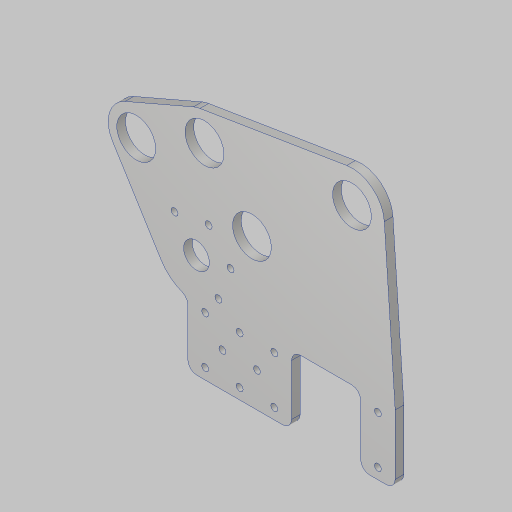
# Autodesk Inventor part: CL3-016
Saved by Autodesk Inventor 2023.5 (Build 275446000, 446)
## iProperties
Created: 2025-01-28
Part Number: CL3-016
Material: Aluminum 6061
Document SubType Name: Modeling
Designer: slick
Density: 2.7 g/cm^3
Appearance: Aluminum - Flat
Mass: 311.171 g
Surface Area: 423.623 cm^2
Volume: 115.249 cm^3
Author: slick
Autodesk Inventor part; units mm, degrees
ref_plane "YZ Plane" through (0, 0, 0) normal (1, 0, 0) x (0, 1, 0)
ref_plane "XZ Plane" through (0, 0, 0) normal (0, 1, 0) x (-1, 0, 0)
ref_plane "XY Plane" through (0, 0, 0) normal (0, 0, 1) x (1, 0, 0)
sketch "Sketch1" plane through (0, 0, 0) normal (0, 0, 1) x (1, 0, 0)
  line L0 (-76.2, 25.4) -> (76.2, 25.4) construction
  line L1 (76.2, 25.4) -> (76.2, -25.4) construction
  line L2 (76.2, -25.4) -> (-76.2, -25.4) construction
  line L3 (-76.2, -25.4) -> (-76.2, 25.4) construction
  line L4 (-76.2, 25.4) -> (76.2, -25.4) construction
  line L5 (76.2, 25.4) -> (-76.2, -25.4) construction
  line L6 (63.5, 17.4625) -> (63.5, -17.4625) construction
  line L7 (9.525, 15.875) -> (41.275, 15.875) construction
  line L8 (41.275, 15.875) -> (41.275, -15.875) construction
  line L9 (41.275, -15.875) -> (9.525, -15.875) construction
  line L10 (9.525, -15.875) -> (9.525, 15.875) construction
  line L11 (9.525, 15.875) -> (41.275, -15.875) construction
  line L12 (41.275, 15.875) -> (9.525, -15.875) construction
  line L13 (76.2, 101.6) -> (187.452, 101.6) construction
  line L14 (187.452, 101.6) -> (187.452, -25.4) construction
  line L15 (187.452, -25.4) -> (76.2, -25.4) construction
  line L16 (76.2, -25.4) -> (76.2, 101.6) construction
  line L17 (76.2, 101.6) -> (187.452, -25.4) construction
  line L18 (187.452, 101.6) -> (76.2, -25.4) construction
  point P0 (0, 0)
  point P1 (63.5, 0)
  point P2 (25.4, 0)
  point P3 (50.8, 0)
  point P4 (0, 0)
  point P5 (9.525, 0)
  point P6 (-12.7, 17.4625)
  point P7 (-12.7, -17.4625)
  point P8 (-25.4, 0)
  point P9 (-38.1, 17.4625)
  point P10 (-38.1, -17.4625)
  point P11 (-50.8, 0)
  point P12 (-63.5, 17.4625)
  point P13 (-63.5, -17.4625)
  point P14 (131.826, 38.1)
  dimension "d0" = 152.4
  dimension "d1" = 50.8
  dimension "d2" = 34.925
  dimension "d3" = 12.7
  dimension "d4" = 31.75
  dimension "d5" = 31.75
  dimension "d6" = 34.925
  dimension "d7" = 25.4
  dimension "d8" = 9.525
  dimension "d9" = 12.7
  dimension "d10" = 12.7
  dimension "d11" = 12.7
  dimension "d12" = 12.7
  dimension "d13" = 12.7
  dimension "d14" = 111.252
  dimension "d15" = 127
  dimension "d16" = 76.2
  constraints: 38 end point, 11 horizontal alignment, 8 midpoint, 6 parallel, 4 vertical alignment, 3 horizontal, 3 perpendicular, 2 coincident, 1 vertical
  measures "d0" distance of L1.end L2.end
  measures "d1" distance of L0.end L1.end
  measures "d2" distance of L6.end L6.start
  measures "d3" distance from line of L1 L6.start
  measures "d4" distance of L8.end L9.end
  measures "d5" distance of L7.end L8.end
  measures "d6" distance between parallel lines of L1 L8
  measures "d7" distance from line of L1 point (50.8, 0)
  measures "d8" distance of point (9.525, 0) point (0, 0)
  measures "d9" horizontal distance of point (0, 0) point (-12.7, 17.463)
  measures "d10" horizontal distance of point (-38.1, 17.463) point (-25.4, 0)
  measures "d11" horizontal distance of point (-38.1, -17.463) point (-50.8, 0)
  measures "d12" horizontal distance of point (-12.7, -17.463) point (-25.4, 0)
  measures "d13" horizontal distance of point (-63.5, 17.463) point (-50.8, 0)
  measures "d14" distance of L14.end L15.end
  measures "d15" distance of L13.end L14.end
  measures "d16" distance between parallel lines of L13 L0
sketch "Sketch2" plane through (0, 0, 0) normal (0, 0, 1) x (1, 0, 0)
  line L0 (63.5, 17.4625) -> (63.5, -17.4625) construction
  line L1 (76.2, 25.4) -> (76.2, -25.4) construction
  line L2 (76.2, -25.4) -> (76.2, 101.6) construction
  line L3 (187.452, -25.4) -> (76.2, -25.4) construction
  line L4 (187.452, 101.6) -> (187.452, -25.4) construction
  line L5 (76.2, 101.6) -> (187.452, -25.4) construction
  line L6 (187.452, 101.6) -> (76.2, -25.4) construction
  line L7 (76.2, 101.6) -> (187.452, 101.6) construction
  line L8 (9.525, 15.875) -> (41.275, 15.875) construction
  line L9 (41.275, 15.875) -> (41.275, -15.875) construction
  line L10 (41.275, -15.875) -> (9.525, -15.875) construction
  line L11 (9.525, -15.875) -> (9.525, 15.875) construction
  line L12 (9.525, 15.875) -> (41.275, -15.875) construction
  line L13 (41.275, 15.875) -> (9.525, -15.875) construction
  line L14 (-76.2, 25.4) -> (76.2, 25.4) construction
  line L15 (76.2, -25.4) -> (-76.2, -25.4) construction
  line L16 (-76.2, 25.4) -> (76.2, -25.4) construction
  line L17 (76.2, 25.4) -> (-76.2, -25.4) construction
  line L18 (-76.2, -25.4) -> (-76.2, 25.4) construction
  line L19 (0, 25.4) -> (0, -25.4)
  line L20 (0, -25.4) -> (-76.2, -25.4)
  line L21 (-76.2, -25.4) -> (-76.2, 25.4)
  line L22 (-76.2, 25.4) -> (25.7652, 154.4619)
  circle A0 centre (44.45, 139.7) radius 14.2875
  circle A1 centre (44.45, 139.7) radius 23.8125 construction
  line L23 (68.2061, 141.338) -> (76.2, 25.4)
  line L24 (76.2, 25.4) -> (76.2, -25.4)
  line L25 (76.2, -25.4) -> (50.8, -25.4)
  line L26 (50.8, -25.4) -> (50.8, 25.4)
  line L27 (50.8, 25.4) -> (0, 25.4)
  arc A2 (68.2061, 141.338) -> (25.7652, 154.4619) centre (44.45, 139.7) ccw
  point P0 (0, 0)
  point P1 (63.5, 0)
  point P2 (131.826, 38.1)
  point P3 (9.525, 0)
  point P4 (0, 0)
  point P5 (25.4, 0)
  point P6 (-63.5, -17.4625)
  point P7 (-63.5, 17.4625)
  point P8 (-50.8, 0)
  point P9 (-38.1, -17.4625)
  point P10 (-38.1, 17.4625)
  point P11 (-25.4, 0)
  point P12 (-12.7, -17.4625)
  point P13 (-12.7, 17.4625)
  point P14 (0, 0)
  point P15 (50.8, 0)
  point P16 (0, 0)
  dimension "d17" = 28.575
  dimension "d18" = 9.525
  dimension "d20" = 9.525
  dimension "d21" = 9.525
  dimension "d31" = 165.1
  dimension "d32" = 19.05
  constraints: 18 end point, 4 point on circle, 3 centre point, 3 coincident, 3 midpoint, 2 collinear, 2 point on line, 2 tangent, 1 perpendicular
  measures "d17" diameter of A0
  measures "d18" radial gap between concentric circles of A0 A1
  measures "d20" distance between parallel lines of L11 L19
  measures "d21" distance between parallel lines of L26 L9
  measures "d31" distance from line of L15 A0.centre
  measures "d32" horizontal distance of point (63.5, 17.463) A0.centre
extrude "Extrusion1" add sketch "Sketch2" along normal blind 6.35
hole "Hole1" at (76.2, 101.6, 0) at (131.826, 38.1, 0) at (187.452, -25.4, 0) at (9.525, 0, 0) at (9.525, 15.875, 0) at (41.275, -15.875, 0) at (41.275, 15.875, 0) at (9.525, -15.875, 0) at (25.4, 0, 0) at (-63.5, -17.4625, 0) at (-63.5, 17.4625, 0) at (-50.8, 0, 0) at (-38.1, -17.4625, 0) at (-38.1, 17.4625, 0) at (-25.4, 0, 0) at (-12.7, -17.4625, 0) at (-12.7, 17.4625, 0) at (63.5, 17.4625, 0) at (63.5, -17.4625, 0) direction (0, 0, 1) diameter 5.1054 end through all clearance for "Flat Head Machine Screw (82)" size "#10" standard "Ansi Unified Screw Threads"
fillet "Fillet1" radius 6.604 7 edges at (50.8, 25.4, 3.175) (0, 25.4, 3.175) (0, -25.4, 3.175) (50.8, -25.4, 3.175) (76.2, -25.4, 3.175) (-76.2, -25.4, 3.175) (-76.2, 25.4, 3.175)
sketch "Sketch4" plane through (0, 0, 6.35) normal (0, 0, 1) x (1, 0, 0)
  circle A0 centre (-69.85, 50.8) radius 25.4 construction
  circle A1 centre (-69.85, 50.8) radius 30.48 construction
  circle A2 centre (-69.85, 50.8) radius 9.525
  circle A3 centre (-69.85, 50.8) radius 6.35 construction
  circle A4 centre (-29.0763, 83.185) radius 45.72 construction
  circle A5 centre (63.5, 17.4625) radius 2.5527 construction
  circle A6 centre (-12.7, -17.4625) radius 2.5527 construction
  circle A7 centre (-38.1, 17.4625) radius 2.5527 construction
  circle A8 centre (-50.8, 0) radius 2.5527 construction
  circle A9 centre (-63.5, -17.4625) radius 2.5527 construction
  circle A10 centre (-63.5, 17.4625) radius 2.5527 construction
  circle A11 centre (-38.1, -17.4625) radius 2.5527 construction
  circle A12 centre (-25.4, 0) radius 2.5527 construction
  circle A13 centre (-12.7, 17.4625) radius 2.5527 construction
  circle A14 centre (63.5, -17.4625) radius 2.5527 construction
  circle A15 centre (44.45, 139.7) radius 14.2875 construction
  arc A16 (68.2061, 141.338) -> (25.7652, 154.4619) centre (44.45, 139.7) ccw construction
  line L0 (68.2061, 141.338) -> (76.2, 25.4) construction
  line L1 (76.2, 25.4) -> (76.2, -18.796) construction
  arc A17 (69.596, -25.4) -> (76.2, -18.796) centre (69.596, -18.796) ccw construction
  line L2 (69.596, -25.4) -> (57.404, -25.4) construction
  arc A18 (50.8, -18.796) -> (57.404, -25.4) centre (57.404, -18.796) ccw construction
  line L3 (50.8, -18.796) -> (50.8, 18.796) construction
  arc A19 (50.8, 18.796) -> (44.196, 25.4) centre (44.196, 18.796) ccw construction
  line L4 (44.196, 25.4) -> (6.604, 25.4) construction
  arc A20 (6.604, 25.4) -> (0, 18.796) centre (6.604, 18.796) ccw construction
  line L5 (0, 18.796) -> (0, -18.796) construction
  arc A21 (-6.604, -25.4) -> (0, -18.796) centre (-6.604, -18.796) ccw construction
  line L6 (-6.604, -25.4) -> (-69.596, -25.4) construction
  arc A22 (-76.2, -18.796) -> (-69.596, -25.4) centre (-69.596, -18.796) ccw construction
  line L7 (-76.2, -18.796) -> (-76.2, 23.106) construction
  arc A23 (-74.7779, 27.2) -> (-76.2, 23.106) centre (-69.596, 23.106) ccw projected
  line L8 (-74.7779, 27.2) -> (25.7652, 154.4619) projected
  line L9 (76.2, -25.4) -> (-127, -25.4) construction
  line L10 (-127, -25.4) -> (-127, 25.4) construction
  line L11 (-127, 25.4) -> (76.2, 25.4) construction
  line L12 (76.2, 25.4) -> (76.2, -25.4) construction
  circle A24 centre (-29.0763, 83.185) radius 14.2875
  arc A25 (61.8711, 140.9012) -> (30.7478, 150.5254) centre (44.45, 139.7) ccw construction
  line L13 (61.8711, 140.9012) -> (69.85, 25.1813) construction
  line L14 (69.85, 25.1813) -> (69.85, -19.05) construction
  line L15 (69.85, -19.05) -> (57.15, -19.05) construction
  line L16 (57.15, -19.05) -> (57.15, 18.796) construction
  arc A26 (57.15, 18.796) -> (44.196, 31.75) centre (44.196, 18.796) ccw construction
  line L17 (44.196, 31.75) -> (6.604, 31.75) construction
  arc A27 (6.604, 31.75) -> (-6.35, 18.796) centre (6.604, 18.796) ccw construction
  line L18 (-6.35, 18.796) -> (-6.35, -19.05) construction
  line L19 (-6.35, -19.05) -> (-69.85, -19.05) construction
  line L20 (-69.85, -19.05) -> (-69.85, 23.1943) construction
  line L21 (-69.85, 23.1943) -> (30.7478, 150.5254) construction
  circle A28 centre (-29.0763, 83.185) radius 12.7 construction
  circle A29 centre (-63.9731, 125.1905) radius 41.91 construction
  circle A30 centre (-63.9731, 125.1905) radius 12.7 construction
  circle A31 centre (-114.13, 103.5909) radius 41.91 construction
  circle A32 centre (-63.9731, 125.1905) radius 14.2875
  circle A33 centre (-114.13, 103.5909) radius 14.2875
  circle A34 centre (-63.9731, 125.1905) radius 20.6375 construction
  circle A35 centre (-114.13, 103.5909) radius 20.6375 construction
  line L22 (-131.6741, 92.723) -> (-95.7613, 34.7489)
  line L23 (-122.2926, 122.5456) -> (-72.1357, 144.1451)
  line L24 (-67.303, 145.5576) -> (40.6078, 163.2005)
  arc A36 (68.2061, 141.338) -> (25.7652, 154.4619) centre (44.45, 139.7) ccw construction
  arc A37 (40.6078, 163.2005) -> (25.7652, 154.4619) centre (44.45, 139.7) ccw
  arc A38 (-122.2926, 122.5456) -> (-131.6741, 92.723) centre (-114.13, 103.5909) ccw
  circle A39 centre (44.45, 139.7) radius 14.2875 construction
  arc A40 (46.5296, 97.3076) -> (27.9705, 178.8135) centre (44.45, 139.7) ccw construction
  circle A41 centre (-63.9731, 125.1905) radius 7.366 construction
  arc A42 (-67.303, 145.5576) -> (-72.1357, 144.1451) centre (-63.9731, 125.1905) ccw
  line L25 (-76.2, 23.106) -> (-76.2, -18.796) construction
  arc A43 (-95.7613, 34.7489) -> (-76.2, 20.9888) centre (-69.85, 50.8) ccw
  line L26 (-76.2, 20.9888) -> (-76.2, 23.106)
  arc A44 (-119.6231, 116.6288) -> (-113.4368, 89.4601) centre (-114.13, 103.5909) ccw construction
  line L27 (27.9705, 178.8135) -> (-119.6231, 116.6288) construction
  line L28 (46.5296, 97.3076) -> (-113.4368, 89.4601) construction
  point P0 (0, 0)
  point P1 (76.2, 3.302)
  point P2 (76.2, 0)
  point P3 (-44.7172, 146.6076)
  point P4 (-73.589, 28.7048)
  point P5 (-44.7862, 54.9187)
  point P6 (-60.885, 74.5653)
  point P7 (-85.9488, 70.4466)
  point P8 (-94.9138, 46.6813)
  point P9 (-78.815, 27.0347)
  point P10 (-53.7512, 31.1534)
  point P11 (-38.81, 72.7262)
  point P12 (-21.1536, 95.0747)
  dimension "d45" = 50.8
  dimension "d46" = 60.96
  dimension "d47" = 19.05
  dimension "d48" = 12.7
  dimension "d49" = 91.44
  dimension "d50" = 6.35
  dimension "d52" = 203.2
  dimension "d53" = 50.8
  dimension "d54" = 76.2
  dimension "d55" = 28.575
  dimension "d56" = 6.35
  dimension "d57" = 25.4
  dimension "d58" = 83.82
  dimension "d59" = 57.785
  dimension "d60" = 25.4
  dimension "d61" = 83.82
  dimension "d62" = 74.3905
  dimension "d64" = 6.35
  dimension "d65" = 6.35
  dimension "d70" = 360
  dimension "d82" = 84.8868
  dimension "d83" = 14.732
  dimension "d86" = 28.2956
  dimension "d92" = 160.1588
  dimension "d93" = 148.1838
  dimension "d94" = 39.4986
  constraints: 38 end point, 25 point on circle, 23 centre point, 15 coincident, 13 tangent, 3 point on line, 2 equal radius, 2 midpoint, 2 parallel, 1 horizontal, 1 horizontal alignment, 1 perpendicular, 1 vertical alignment, 21 other
  measures "d46" diameter of A1
  measures "d47" diameter of A2
  measures "d48" diameter of A3
  measures "d49" diameter of A4
  measures "d50" distance from line of L7 point (-69.85, 50.8)
  measures "d52" distance of L10.end L11.end
  measures "d53" distance of L9.end L10.end
  measures "d54" distance from line of L9 point (-69.85, 50.8)
  measures "d55" diameter of A24
  measures "d56" distance between parallel lines of L8 L21
  measures "d57" diameter of A28
  measures "d58" diameter of A29
  measures "d59" distance from line of L4 A4.centre
  measures "d60" diameter of A30
  measures "d61" diameter of A31
  measures "d62" vertical distance of point (-69.85, 50.8) A29.centre
  measures "d64" radial gap between concentric circles of A32 A34
  measures "d65" radial gap between concentric circles of A33 A35
  measures "d82" diameter of A40
  measures "d83" diameter of A41
  measures "d86" diameter of A44
  measures "d92" distance of L27.start L27.end
extrude "Extrusion3" add sketch "Sketch4" against normal up to surface (6.35 mm away) contours A23 L26 A43 L22 A38 L23 A42 L24 A37 L8 A24
extrude "Extrusion4" cut sketch "Sketch4" against normal through all contours A2 | A24 L8 | L8 A24
hole "Hole2" at (-44.7862, 54.9187, 6.35) at (-60.885, 74.5653, 6.35) at (-85.9488, 70.4466, 6.35) at (-53.7512, 31.1534, 6.35) direction (0, 0, -1) diameter 5.1054 end through all clearance for "Flat Head Machine Screw (82)" size "#10" standard "Ansi Unified Screw Threads"
fillet "Fillet4" radius 6.604 1 edges at (-76.2, 20.9888, 3.175)
equation "\"off\" = 6.35"
body "Solid1"
